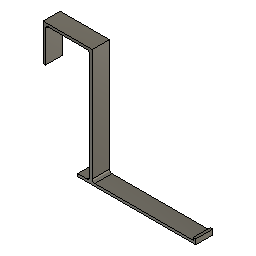
POT-HANGER (Autodesk Fusion 360 design; units mm, degrees)
Autodesk Fusion 360 part; units mm, degrees
sketch "Sketch1" plane through (0, 0, 0) normal (0, 1, 0) x (1, 0, 0)
  line L0 (0, 0) -> (0, -3)
  line L1 (0, -3) -> (14, -3)
  line L2 (14, -3) -> (14, -134)
  line L3 (14, -134) -> (-37.5, -134)
  line L4 (-37.5, -134) -> (-37.5, -94)
  line L5 (-37.5, -94) -> (-40.5, -94)
  line L6 (-40.5, -94) -> (-40.5, -137)
  line L7 (-40.5, -137) -> (17, -137)
  line L8 (17, -137) -> (17, -3)
  line L9 (17, -3) -> (135, -3)
  line L10 (135, -3) -> (135, -6)
  line L11 (135, -6) -> (138, -6)
  line L12 (138, -6) -> (138, 0)
  line L13 (138, 0) -> (0, 0)
  dimension "d1" = 3
  dimension "d2" = 51.5
  dimension "d3" = 3
  dimension "d4" = 3
  dimension "d5" = 3
  dimension "d6" = 3
  dimension "d7" = 3
  dimension "d8" = 14
  dimension "d9" = 135
  dimension "d10" = 3
  dimension "d11" = 131
  dimension "d12" = 40
  constraint coincident L0.start L13.end
  constraint vertical L0
  constraint perpendicular L0 L1
  constraint perpendicular L1 L2
  constraint perpendicular L2 L3
  constraint perpendicular L3 L4
  constraint perpendicular L4 L5
  constraint perpendicular L3 L6
  constraint perpendicular L6 L7
  constraint perpendicular L7 L8
  constraint perpendicular L8 L9
  constraint perpendicular L9 L10
  constraint perpendicular L10 L11
  constraint perpendicular L11 L12
  constraint perpendicular L0 L13
  measures "d1" distance of L4.end L5.end
  measures "d2" distance of L2.end L3.end
  measures "d3" distance of L3 L7
  measures "d4" distance of L2 L8
  measures "d5" distance of L10.end L11.end
  measures "d6" distance of L0.start L0.end
  measures "d7" distance of L9 L13
  measures "d8" distance of L0 L2
  measures "d9" distance of L0 L10
  measures "d10" distance of L9 L11
  measures "d11" distance of L3 L9
  measures "d12" distance of L3 L5.end
extrude "Extrude1" add sketch "Sketch1" along normal blind 20
fillet "Fillet1" radius 3 1 edges at (-37.5, 10, 134)
fillet "Fillet2" radius 3 1 edges at (14, 10, 134)
fillet "Fillet3" radius 3 1 edges at (14, 10, 3)
fillet "Fillet4" radius 3 1 edges at (17, 10, 3)
